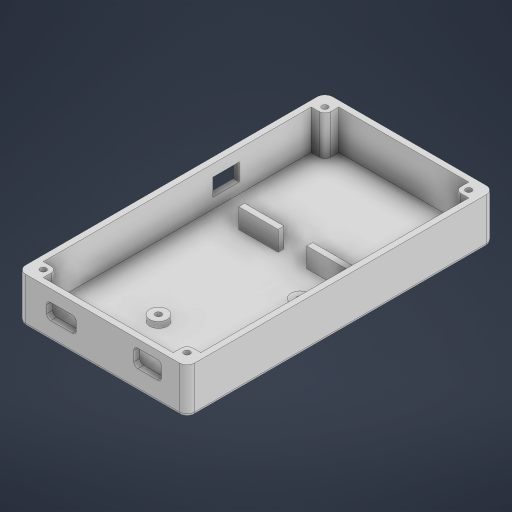
# Autodesk Inventor part: CASING NEW
Saved by Autodesk Inventor 2024 (Build 280153000, 153)
## iProperties
Created: 2025-06-22
Part Number: CASING NEW
Material: Generic
Document SubType Name: Modeling
Designer: ASUS
Density: 1 g/cm^3
Appearance: Default
Author: ASUS
Autodesk Inventor part; units mm, degrees
ref_plane "YZ Plane" through (0, 0, 0) normal (1, 0, 0) x (0, 1, 0)
ref_plane "XZ Plane" through (0, 0, 0) normal (0, 1, 0) x (-1, 0, 0)
ref_plane "XY Plane" through (0, 0, 0) normal (0, 0, 1) x (1, 0, 0)
sketch "Sketch1" plane through (0, 0, 0) normal (0, 1, 0) x (-1, 0, 0)
  line L0 (-43, -78) -> (43, -78)
  line L1 (43, -78) -> (43, 78)
  line L2 (43, 78) -> (-43, 78)
  line L3 (-43, 78) -> (-43, -78)
  point P0 (0, 0)
  constraints: 8 end point, 2 parallel, 1 perpendicular
extrude "Extrusion1" add sketch "Sketch1" along normal blind 3
sketch "Sketch2" plane through (0, 3, 0) normal (0, 1, 0) x (1, 0, 0)
  line L0 (-33, 75) -> (33, 75)
  line L1 (40, 68) -> (40, -68)
  line L2 (33, -75) -> (-33, -75)
  line L3 (-40, -68) -> (-40, 68)
  line L4 (-40, 75) -> (40, -75) construction
  line L5 (40, 75) -> (-40, -75) construction
  line L6 (43, 78) -> (-43, 78)
  line L7 (-43, 78) -> (-43, -78)
  line L8 (-43, -78) -> (43, -78)
  line L9 (43, -78) -> (43, 78)
  line L10 (-40, 75) -> (-33, 75)
  line L11 (-33, 75) -> (-33, 71)
  line L12 (-36, 68) -> (-40, 68)
  line L13 (-40, 68) -> (-40, 75)
  circle A0 centre (-36.5, 71.5) radius 1.5
  arc A1 (-36, 68) -> (-33, 71) centre (-36, 71) ccw
  line L14 (40, 75) -> (-40, -75) construction
  line L15 (33, 75) -> (33, 71)
  line L16 (36, 68) -> (40, 68)
  circle A2 centre (36.5, 71.5) radius 1.5
  arc A3 (33, 71) -> (36, 68) centre (36, 71) ccw
  line L17 (-40, -75) -> (40, 75) construction
  line L18 (-33, -75) -> (-33, -71)
  line L19 (-36, -68) -> (-40, -68)
  circle A4 centre (-36.5, -71.5) radius 1.5
  arc A5 (-33, -71) -> (-36, -68) centre (-36, -71) ccw
  line L20 (36, -68) -> (40, -68)
  arc A6 (36, -68) -> (33, -71) centre (36, -71) ccw
  circle A7 centre (36.5, -71.5) radius 1.5
  line L21 (33, -75) -> (33, -71)
  point P0 (0, 0)
  point P1 (-33, 68)
  point P2 (33, 68)
  point P3 (-33, -68)
  dimension "d5" = 80
  dimension "d6" = 150
  dimension "d7" = 3
  dimension "d42" = 7
  dimension "d43" = 7
  dimension "d45" = 3
  dimension "d46" = 3
  constraints: 44 end point, 8 centre point, 8 point on circle, 6 parallel, 6 point on line, 3 perpendicular, 2 horizontal, 2 midpoint, 2 tangent
  measures "d5" distance of L4.end L5.end
  measures "d6" distance of L5.start L4.end
  measures "d7" distance between parallel lines of L0 L6
  measures "d42" distance of L3.end point (-33, 68)
  measures "d43" distance of L0.start point (-33, 68)
  measures "d45" diameter of A0
  measures "d46" radius of A1
extrude "Extrusion2" add sketch "Sketch2" along normal blind 20 contours L11 A1 L12 L13 L10 | L9 L8 L7 L6
fillet "Fillet1" radius 4 4 edges at (-43, 11.5, 78) (43, 11.5, 78) (43, 11.5, -78) (-43, 11.5, -78)
sketch "Sketch3" plane through (0, 3, 0) normal (0, 1, 0) x (1, 0, 0)
  line L0 (-4.5882, 18.801) -> (-4.5882, 15.801)
  line L1 (-24.5882, 18.801) -> (-24.5882, 15.801)
  line L2 (10, 18.801) -> (10, 15.801)
  line L3 (-24.5882, 18.801) -> (-4.5882, 18.801)
  line L4 (-24.5882, 15.801) -> (-4.5882, 15.801)
  line L5 (10, 18.801) -> (30, 18.801)
  line L6 (10, 15.801) -> (30, 15.801)
  line L7 (30, 18.801) -> (38.3417, 18.801)
  line L8 (30, 15.801) -> (38.3417, 15.801)
  line L9 (38.3417, 18.801) -> (38.3417, 15.801)
  point P0 (0, 0)
  constraints: 20 end point, 4 parallel, 3 horizontal, 1 perpendicular
extrude "Extrusion3" add sketch "Sketch3" along normal blind 10
sketch "Sketch6" plane through (0, 3, 0) normal (0, 1, 0) x (1, 0, 0)
  line L0 (-33, -75) -> (33, -75) projected
  line L1 (-40, 68) -> (-40, -68) projected
  line L2 (0, -75) -> (0, -69.5874)
  circle A0 centre (-4.6, -44.9) radius 1.5
  circle A1 centre (-4.6, -44.9) radius 4.5
  circle A2 centre (24.2, -1.9) radius 1.5
  circle A3 centre (24.2, -1.9) radius 4.5
  point P0 (0, 0)
  constraints: 4 centre point, 2 end point, 1 midpoint, 1 vertical
extrude "Extrusion5" add sketch "Sketch6" along normal blind 3
sketch "Sketch7" plane through (-43, 0, -74) normal (-1, 0, 0) x (0, 0, 1)
  line L0 (0, 23) -> (0, 0) projected
  line L1 (42.5, 8.3188) -> (56, 8.3188)
  line L2 (56, 8.3188) -> (56, 17.1188)
  line L3 (56, 17.1188) -> (42.5, 17.1188)
  line L4 (42.5, 17.1188) -> (42.5, 8.3188)
  line L5 (42.5, 8.3188) -> (56, 17.1188) construction
  line L6 (56, 8.3188) -> (42.5, 17.1188) construction
  point P0 (74, 0)
  dimension "d58" = 13.5
  dimension "d59" = 8.8
  constraints: 12 end point, 2 parallel, 1 horizontal, 1 perpendicular
  measures "d58" distance of L3.end L2.end
  measures "d59" distance of L2.end L1.end
extrude "Extrusion6" cut sketch "Sketch7" against normal blind 3
sketch "Sketch8" plane through (-39, 0, 78) normal (0, 0, 1) x (1, 0, 0)
  line L0 (12.7606, 17) -> (23.7606, 17)
  line L1 (25.7606, 15) -> (25.7606, 11)
  line L2 (23.7606, 9) -> (12.7606, 9)
  line L3 (10.7606, 11) -> (10.7606, 15)
  arc A0 (12.7606, 17) -> (10.7606, 15) centre (12.7606, 15) ccw
  arc A1 (25.7606, 15) -> (23.7606, 17) centre (23.7606, 15) ccw
  arc A2 (23.7606, 9) -> (25.7606, 11) centre (23.7606, 11) ccw
  arc A3 (10.7606, 11) -> (12.7606, 9) centre (12.7606, 11) ccw
  line L4 (82, 23) -> (82, 0) projected
  line L5 (78, 0) -> (0, 0) projected
  line L6 (71.3066, 0) -> (87.3066, 0) construction
  line L7 (72, 3) -> (72, 23) projected
  line L8 (72, 11.5) -> (81, 11.5) construction
  line L9 (49, 13) -> (77.3417, 13) projected
  line L10 (57, 19) -> (67, 19)
  line L11 (69, 17) -> (69, 12)
  line L12 (67, 10) -> (57, 10)
  line L13 (55, 12) -> (55, 17)
  line L14 (55, 19) -> (69, 10) construction
  line L15 (69, 19) -> (55, 10) construction
  line L16 (0, 23) -> (78, 23) projected
  arc A4 (57, 19) -> (55, 17) centre (57, 17) ccw
  arc A5 (55, 12) -> (57, 10) centre (57, 12) ccw
  arc A6 (69, 17) -> (67, 19) centre (67, 17) ccw
  arc A7 (67, 10) -> (69, 12) centre (67, 12) ccw
  point P0 (39, 0)
  point P1 (25.7606, 9)
  point P2 (25.7606, 17)
  point P3 (10.7606, 9)
  point P4 (69, 13)
  dimension "d68" = 15
  dimension "d69" = 8
  dimension "d70" = 2
  dimension "d98" = 14
  dimension "d99" = 4
  dimension "d100" = 9
  dimension "d101" = 2
  dimension "d102" = 2
  dimension "d103" = 2
  dimension "d104" = 2
  dimension "d105" = 13
  dimension "d106" = 6
  constraints: 24 end point, 16 point on circle, 16 tangent, 15 point on line, 8 centre point, 4 horizontal, 4 parallel, 3 equal radius, 2 perpendicular
  measures "d68" distance of point (25.761, 9) point (10.761, 9)
  measures "d69" distance of point (25.761, 17) point (25.761, 9)
  measures "d70" radius of A0
  measures "d98" distance of L14.end L15.end
  measures "d99" distance between parallel lines of L10 L16
  measures "d100" distance of L15.start L14.end
  measures "d101" radius of A4
  measures "d102" radius of A5
  measures "d103" radius of A6
  measures "d104" radius of A7
  measures "d105" distance between parallel lines of L11 L4
  measures "d106" distance between parallel lines of L0 L16
extrude "Extrusion7" cut sketch "Sketch8" against normal blind 3
fillet "Fillet3" radius 1.5 8 edges at (-41.8284, 0, 76.8284) (0, 0, 78) (41.8284, 0, 76.8284) (43, 0, 0) (41.8284, 0, -76.8284) (0, 0, -78) (-41.8284, 0, -76.8284) (-43, 0, 0)
body "Solid1"
